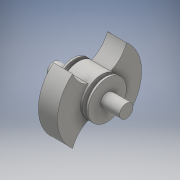
# Autodesk Inventor part: arma
Saved by Autodesk Inventor 2016 (Build 200138000, 138)
## iProperties
Created: 2019-03-15
Part Number: arma
Material: Genérico
Document SubType Name: Modeling
Designer: FIMCP
Density: 1 g/cm^3
Appearance: Valor por defecto
Author: FIMCP
Autodesk Inventor part; units mm, degrees
ref_plane "YZ Plane" through (0, 0, 0) normal (1, 0, 0) x (0, 1, 0)
ref_plane "XZ Plane" through (0, 0, 0) normal (0, 1, 0) x (-1, 0, 0)
ref_plane "XY Plane" through (0, 0, 0) normal (0, 0, 1) x (1, 0, 0)
sketch "Boceto1" plane through (0, 0, 0) normal (1, 0, 0) x (0, 1, 0)
  circle A0 centre (0, 0) radius 3.5
  dimension "d0" = 7
  constraints: 1 centre point, 1 coincident
  measures "d0" diameter of A0
extrude "Extrusión1" add sketch "Boceto1" along normal mid plane 38
sketch "Boceto2" plane through (0, 0, 0) normal (1, 0, 0) x (0, 1, 0)
  arc A0 (14.1014, -16.8864) -> (-14.1014, -16.8864) centre (0, -22) ccw
  arc A1 (-14.1014, 16.8864) -> (14.1014, 16.8864) centre (0, 22) ccw
  arc A2 (-14.1014, 16.8864) -> (-14.1014, -16.8864) centre (0, 0) ccw
  arc A3 (14.1014, -16.8864) -> (14.1014, 16.8864) centre (0, 0) ccw
  dimension "d4" = 30
  dimension "d5" = 30
  constraints: 8 point on circle, 4 centre point, 1 coincident
  measures "d4" diameter of A0
  measures "d5" diameter of A1
extrude "Extrusión2" add sketch "Boceto2" along normal mid plane 10
sketch "Boceto3" plane through (0, 0, 0) normal (1, 0, 0) x (0, 1, 0)
  circle A0 centre (0, 0) radius 10
  dimension "d8" = 20
  constraints: 1 centre point, 1 coincident
  measures "d8" diameter of A0
extrude "Extrusión3" add sketch "Boceto3" along normal mid plane 12
sketch "Boceto4" plane through (0, 0, 0) normal (1, 0, 0) x (0, 1, 0)
  circle A0 centre (0, 0) radius 3.5 projected
  circle A1 centre (0, 0) radius 7
  dimension "d11" = 14
  constraints: 1 centre point, 1 coincident
  measures "d11" diameter of A1
extrude "Extrusión4" add sketch "Boceto4" along normal mid plane 18
sketch "Boceto6" plane through (0, 0, 0) normal (0, 1, 0) x (-1, 0, 0)
  line L0 (9, -3.5) -> (9, 3.5) projected
  line L1 (9, 0) -> (8, 0)
  line L2 (8, 0) -> (8, -10)
  line L3 (8, -10) -> (9, -10)
  line L4 (9, -10) -> (9, 0)
  line L5 (26.6, 0) -> (-26.6, 0) projected
  point P0 (0, 0)
  dimension "d15" = 1
  dimension "d16" = 10
  constraints: 8 end point, 2 parallel, 1 horizontal, 1 midpoint, 1 perpendicular
  measures "d15" distance of L3.end L2.end
  measures "d16" distance of L2.end L1.end
revolve "Revolución1" add sketch "Boceto6" angle 360 about axis through (-10, 0, 0) along (1, 0, 0)
sketch "Boceto7" plane through (0, 0, 0) normal (0, 1, 0) x (-1, 0, 0)
  line L0 (-9, 7) -> (-9, -7) projected
  line L1 (-9, 0) -> (-8, 0)
  line L2 (-8, 0) -> (-8, -10)
  line L3 (-8, -10) -> (-9, -10)
  line L4 (-9, -10) -> (-9, 0)
  line L5 (26.6, 0) -> (-26.6, 0) projected
  point P0 (0, 0)
  dimension "d18" = 1
  dimension "d19" = 10
  constraints: 8 end point, 2 parallel, 1 horizontal, 1 midpoint, 1 perpendicular
  measures "d18" distance of L2.end L3.end
  measures "d19" distance of L1.end L2.end
revolve "Revolución2" add sketch "Boceto7" angle 360 about axis through (-10, 0, 0) along (1, 0, 0)
